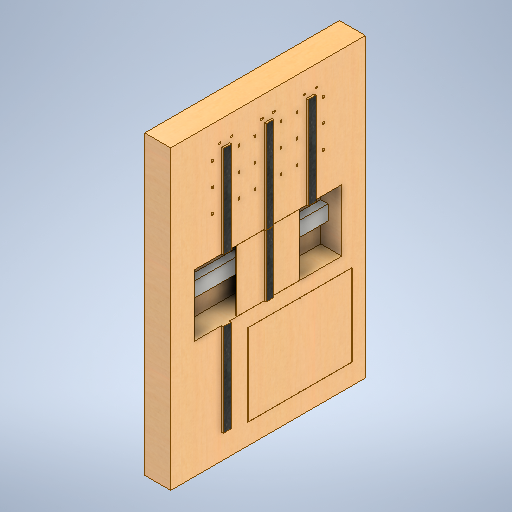
# Autodesk Inventor part: 3D cely
Saved by Autodesk Inventor 2025.1 (Build 291241000, 241)
## iProperties
Created: 2024-11-03
Part Number: 3D cely
Material: ABS plast
Document SubType Name: Sheet Metal
Designer: nelan
Density: 1.06 g/cm^3
Appearance: Borovice těžká – masiv světle obarvený – nízký lesk
Sheet Metal Rule: Výchozí
Author: nelan
Autodesk Inventor part; units mm, degrees
ref_plane "YZ Plane" through (0, 0, 0) normal (1, 0, 0) x (0, 1, 0)
ref_plane "XZ Plane" through (0, 0, 0) normal (0, 1, 0) x (-1, 0, 0)
ref_plane "XY Plane" through (0, 0, 0) normal (0, 0, 1) x (1, 0, 0)
sketch "Náčrt1" plane through (0, 0, 0) normal (1, 0, 0) x (0, 1, 0)
  line L0 (-400, -262.5) -> (400, -262.5)
  line L1 (400, -262.5) -> (400, 262.5)
  line L2 (-400, 262.5) -> (-400, -262.5)
  line L3 (-400, -262.5) -> (400, 262.5) construction
  line L4 (400, -262.5) -> (-400, 262.5) construction
  line L5 (-400, -262.5) -> (-320, -262.5)
  line L6 (-320, -262.5) -> (-320, -258.5)
  line L7 (-320, -258.5) -> (-400, -258.5)
  line L8 (-400, -258.5) -> (-400, -262.5)
  line L9 (-240, -258.5) -> (-240, -262.5)
  line L10 (-240, -258.5) -> (-160, -258.5)
  line L11 (-160, -258.5) -> (-160, -262.5)
  line L12 (-80, -258.5) -> (0, -258.5)
  line L13 (0, -258.5) -> (0, -262.5)
  line L14 (-80, -258.5) -> (-80, -262.5)
  line L15 (80, -258.5) -> (80, -262.5)
  line L16 (80, -258.5) -> (160, -258.5)
  line L17 (160, -258.5) -> (160, -262.5)
  line L18 (240, -258.5) -> (240, -262.5)
  line L19 (240, -258.5) -> (320, -258.5)
  line L20 (320, -258.5) -> (320, -262.5)
  line L21 (-400, 262.5) -> (400, 262.5)
  line L22 (-396, -258.5) -> (-400, -258.5)
  line L23 (-396, -258.5) -> (-400, -258.5)
  line L24 (-320, 258.5) -> (-240, 258.5)
  line L25 (-160, 258.5) -> (-80, 258.5)
  line L26 (0, 258.5) -> (80, 258.5)
  line L27 (160, 258.5) -> (240, 258.5)
  line L28 (320, 258.5) -> (400, 258.5)
  line L29 (320, 258.5) -> (320, 262.5)
  line L30 (240, 258.5) -> (240, 262.5)
  line L31 (160, 258.5) -> (160, 262.5)
  line L32 (80, 258.5) -> (80, 262.5)
  line L33 (0, 258.5) -> (0, 262.5)
  line L34 (-80, 258.5) -> (-80, 262.5)
  line L35 (-160, 258.5) -> (-160, 262.5)
  line L36 (-240, 258.5) -> (-240, 262.5)
  line L37 (-320, 258.5) -> (-320, 262.5)
  line L38 (400, 258.5) -> (396, 258.5)
  line L39 (396, 206.4) -> (396, 154.3)
  line L40 (396, 102.2) -> (396, 50.1)
  line L41 (396, -2) -> (396, -54.1)
  line L42 (396, -106.2) -> (396, -158.3)
  line L43 (396, -210.4) -> (396, -262.5)
  line L44 (-396, 262.5) -> (-396, 210.4)
  line L45 (-396, 210.4) -> (-400, 210.4)
  line L46 (-396, 158.3) -> (-396, 106.2)
  line L47 (-396, 54.1) -> (-396, 2)
  line L48 (-396, -50.1) -> (-396, -102.2)
  line L49 (-396, -154.3) -> (-396, -206.4)
  line L50 (-396, 158.3) -> (-400, 158.3)
  line L51 (-396, 106.2) -> (-400, 106.2)
  line L52 (-396, 54.1) -> (-400, 54.1)
  line L53 (-396, 2) -> (-400, 2)
  line L54 (-396, -50.1) -> (-400, -50.1)
  line L55 (-396, -102.2) -> (-400, -102.2)
  line L56 (-396, -154.3) -> (-400, -154.3)
  line L57 (-396, -206.4) -> (-400, -206.4)
  line L58 (396, 206.4) -> (400, 206.4)
  line L59 (396, 154.3) -> (400, 154.3)
  line L60 (396, 102.2) -> (400, 102.2)
  line L61 (396, 50.1) -> (400, 50.1)
  line L62 (396, -2) -> (400, -2)
  line L63 (396, -54.1) -> (400, -54.1)
  line L64 (396, -106.2) -> (400, -106.2)
  line L65 (396, -158.3) -> (400, -158.3)
  line L66 (396, -210.4) -> (400, -210.4)
  line L67 (396, -262.5) -> (400, -262.5)
  point P0 (0, 0)
  dimension "d0" = 800
  dimension "d1" = 525
  dimension "d4" = 80
  dimension "d5" = 4
  dimension "d7" = 80
  dimension "d9" = 80
  dimension "d11" = 80
  dimension "d13" = 80
  dimension "d14" = 4
  dimension "d15" = 4
  dimension "d16" = 4
  dimension "d17" = 4
  dimension "d18" = 4
  dimension "d19" = 4
  dimension "d20" = 80
  dimension "d21" = 80
  dimension "d22" = 80
  dimension "d40" = 80
  dimension "d41" = 80
  dimension "d42" = 80
  dimension "d43" = 80
  dimension "d44" = 80
  dimension "d45" = 80
  dimension "d46" = 80
  dimension "d47" = 80
  dimension "d48" = 80
  dimension "d49" = 4
  dimension "d50" = 4
  dimension "d51" = 52.1
  dimension "d52" = 52.1
  dimension "d53" = 52.1
  dimension "d54" = 52.1
  dimension "d55" = 52.1
  dimension "d56" = 52.1
  dimension "d57" = 52.1
  dimension "d58" = 52.1
  dimension "d59" = 52.1
  dimension "d60" = 52.1
  dimension "d67" = 52.1
  dimension "d68" = 52.1
  dimension "d69" = 52.1
  dimension "d70" = 52.1
  dimension "d71" = 52.1
  dimension "d72" = 52.1
  dimension "d73" = 52.1
  dimension "d74" = 52.1
  dimension "d75" = 52.1
  dimension "d76" = 52.1
  dimension "d77" = 4
  dimension "d78" = 4
  dimension "d79" = 4
  dimension "d80" = 4
  dimension "d81" = 4
  dimension "d82" = 4
  dimension "d83" = 4
  dimension "d84" = 4
  dimension "d85" = 4
  constraints: 128 end point, 20 horizontal, 16 vertical, 12 point on line, 9 vertical alignment, 6 horizontal alignment, 4 parallel, 2 midpoint, 2 perpendicular, 1 coincident, 50 other
  measures "d0" distance of L4.end L3.end
  measures "d1" distance of L3.end L4.start
  measures "d4" distance of L7.end L6.end
  measures "d5" distance of L6.end L5.end
  measures "d7" distance of L9.start L10.end
  measures "d9" distance of L12.start L12.end
  measures "d11" distance of L15.start L16.end
  measures "d13" distance of L18.start L19.end
  measures "d14" distance of L9.end L9.start
  measures "d15" distance of L11.end L10.end
  measures "d16" distance of L13.end L12.end
  measures "d17" distance of L17.end L16.end
  measures "d18" distance of L18.end L18.start
  measures "d19" distance of L20.end L19.end
  measures "d20" distance of L4.start L20.end
  measures "d21" distance of L18.end L17.end
  measures "d22" distance of L11.end L14.end
  measures "d40" distance of L24.start L24.end
  measures "d41" distance of L24.end L25.start
  measures "d42" distance of L25.start L25.end
  measures "d43" distance of L25.end L26.start
  measures "d44" distance of L26.start L26.end
  measures "d45" distance of L26.end L27.start
  measures "d46" distance of L27.start L27.end
  measures "d47" distance of L27.end L28.start
  measures "d48" distance of L28.start L28.end
  measures "d49" distance of L24.start L37.end
  measures "d50" distance of L28.end L38.end
  measures "d51" distance of L38.end L39.start
  measures "d52" distance of L39.start L39.end
  measures "d53" distance of L39.end L40.start
  measures "d54" distance of L40.start L40.end
  measures "d55" distance of L40.end L41.start
  measures "d56" distance of L41.start L41.end
  measures "d57" distance of L41.end L42.start
  measures "d58" distance of L42.start L42.end
  measures "d59" distance of L42.end L43.start
  measures "d60" distance of L43.start L43.end
  measures "d67" distance of L44.start L44.end
  measures "d68" distance of L44.end L46.start
  measures "d69" distance of L46.start L46.end
  measures "d70" distance of L46.end L47.start
  measures "d71" distance of L47.start L47.end
  measures "d72" distance of L47.end L48.start
  measures "d73" distance of L48.start L48.end
  measures "d74" distance of L48.end L49.start
  measures "d75" distance of L49.start L49.end
  measures "d76" distance of L49.end L22.start
  measures "d81" distance of L43.start L66.end
  measures "d82" distance of L42.end L65.end
  measures "d83" distance of L41.end L63.end
  measures "d84" distance of L40.end L61.end
  measures "d85" distance of L39.end L59.end
extrude "Vysunutí2" add sketch "Náčrt1" against normal blind 4 contours L6 L7 L2 L57 L49 L56 L55 L48 L54 L53 L47 L52 L51 L46 L50 L45 L44 L21 L37 L24 L36 L35 L25 L34 L33 L26 L32 L31 L27 L30 L29 L28 L1 L58 L39 L59 L60 L40 L61 L62 L41 L63 L64 L42 L65 L66 L43 L0 L20 L19 L18 L17 L16 L15 L13 L12 L14 L11 L10 L9
sketch "Náčrt4" plane through (0, -240, -258.5) normal (0, 0, -1) x (-1, 0, 0)
  line L0 (0, -160) -> (4, -160) projected
  line L1 (0, -160) -> (70, -160)
  line L2 (70, -160) -> (70, 640)
  line L3 (70, 640) -> (0, 640)
  line L4 (0, 640) -> (0, -160)
  line L5 (57, -64) -> (65, -64)
  line L6 (65, -64) -> (65, 16)
  line L7 (65, 16) -> (57, 16)
  line L8 (57, 16) -> (57, -64)
  line L9 (65, 112) -> (57, 112)
  line L10 (57, 112) -> (57, 192)
  line L11 (57, 192) -> (65, 192)
  line L12 (65, 192) -> (65, 112)
  line L13 (57, 288) -> (65, 288)
  line L14 (65, 288) -> (65, 368)
  line L15 (65, 368) -> (57, 368)
  line L16 (57, 368) -> (57, 288)
  line L17 (65, 544) -> (57, 544)
  line L18 (57, 544) -> (57, 464)
  line L19 (57, 464) -> (65, 464)
  line L20 (65, 464) -> (65, 544)
  point P0 (0, 240)
  dimension "d88" = 70
  dimension "d89" = 800
  dimension "d90" = 8
  dimension "d91" = 80
  dimension "d92" = 8
  dimension "d93" = 80
  dimension "d94" = 8
  dimension "d95" = 80
  dimension "d96" = 8
  dimension "d97" = 80
  dimension "d98" = 96
  dimension "d99" = 96
  dimension "d100" = 96
  dimension "d101" = 96
  dimension "d102" = 5
  dimension "d103" = 5
  dimension "d104" = 5
  constraints: 40 end point, 10 parallel, 5 horizontal, 5 perpendicular, 1 point on line
  measures "d88" distance of L3.end L2.end
  measures "d89" distance of L2.end L1.end
  measures "d90" distance of L7.end L6.end
  measures "d91" distance of L6.end L5.end
  measures "d92" distance of L10.end L11.end
  measures "d93" distance of L9.end L10.end
  measures "d94" distance of L15.end L14.end
  measures "d95" distance of L14.end L13.end
  measures "d96" distance of L19.end L18.end
  measures "d97" distance of L18.end L17.end
  measures "d98" vertical distance of L5.end L1.end
  measures "d99" vertical distance of L2.end L17.end
  measures "d100" distance of L18.end L15.end
  measures "d101" distance of L13.start L10.end
  measures "d102" distance between parallel lines of L2 L6
  measures "d103" distance between parallel lines of L2 L12
  measures "d104" distance between parallel lines of L2 L20
extrude "Vysunutí3" add sketch "Náčrt4" along normal blind 4
sketch "Náčrt5" plane through (0, -396, 2) normal (0, -1, 0) x (1, 0, 0)
  line L0 (-70, -260.5) -> (-70, -264.5) projected
  line L1 (0, 260.5) -> (-70, 260.5)
  line L2 (-70, 260.5) -> (-70, -264.5)
  line L3 (-70, -264.5) -> (0, -264.5)
  line L4 (0, -264.5) -> (0, 260.5)
  line L5 (-57, 187.25) -> (-65, 187.25)
  line L6 (-65, 187.25) -> (-65, 107.25)
  line L7 (-65, 107.25) -> (-57, 107.25)
  line L8 (-57, 107.25) -> (-57, 187.25)
  line L9 (-57, 40) -> (-65, 40)
  line L10 (-65, 40) -> (-65, -40)
  line L11 (-65, -40) -> (-57, -40)
  line L12 (-57, -40) -> (-57, 40)
  line L13 (-57, -111.25) -> (-65, -111.25)
  line L14 (-65, -111.25) -> (-65, -191.25)
  line L15 (-65, -191.25) -> (-57, -191.25)
  line L16 (-57, -191.25) -> (-57, -111.25)
  line L17 (0, 0) -> (-4, 0) projected
  line L18 (-4, -260.5) -> (-70, -260.5) projected
  point P0 (0, -2)
  point P1 (-57, 0)
  point P2 (-2, 0)
  dimension "d107" = 70
  dimension "d108" = 525
  dimension "d109" = 8
  dimension "d110" = 80
  dimension "d111" = 8
  dimension "d112" = 80
  dimension "d113" = 8
  dimension "d114" = 80
  dimension "d115" = 5
  dimension "d116" = 5
  dimension "d117" = 73.25
  dimension "d118" = 69.25
  constraints: 32 end point, 8 parallel, 4 horizontal, 4 perpendicular, 2 midpoint, 1 horizontal alignment, 1 point on line
  measures "d107" distance of L0.end L3.end
  measures "d108" distance of L1.end L0.end
  measures "d109" distance of L7.end L6.end
  measures "d110" distance of L6.end L5.end
  measures "d111" distance of L11.end L10.end
  measures "d112" distance of L10.end L9.end
  measures "d113" distance of L15.end L14.end
  measures "d114" distance of L14.end L13.end
  measures "d115" distance between parallel lines of L2 L10
  measures "d116" distance between parallel lines of L2 L6
  measures "d117" vertical distance of L5.start L1.end
  measures "d118" distance from line of L18 L15.end
mirror "Zrcadlit1" about plane through (0, 0, 0) normal (0, 0, 1) of "Vysunutí3"
extrude "Vysunutí4" add sketch "Náčrt5" along normal blind 4
mirror "Zrcadlit2" about plane through (0, 0, 0) normal (0, 1, 0) of "Vysunutí4"
sketch "Náčrt6" plane through (0, 0, 0) normal (1, 0, 0) x (0, 0, -1)
  line L0 (-199, 83.5) -> (199, 83.5)
  line L1 (199, 83.5) -> (199, -83.5)
  line L2 (199, -83.5) -> (-199, -83.5)
  line L3 (-199, -83.5) -> (-199, 83.5)
  line L4 (-199, 83.5) -> (199, -83.5) construction
  line L5 (199, 83.5) -> (-199, -83.5) construction
  point P0 (0, 0)
  dimension "d121" = 398
  dimension "d122" = 167
  constraints: 12 end point, 2 midpoint, 2 parallel, 1 horizontal, 1 perpendicular
  measures "d121" distance of L1.end L2.end
  measures "d122" distance of L0.end L1.end
extrude "Vysunutí5" cut sketch "Náčrt6" against normal blind 4
sketch "Náčrt7" plane through (0, 83.5, -199) normal (0, -1, 0) x (1, 0, 0)
  line L0 (-57, 0) -> (-4, 0)
  line L1 (-4, 398) -> (-57, 398)
  line L2 (-57, 398) -> (-57, 0)
  line L3 (-4, 398) -> (-4, 0)
  line L4 (-4, 457.5) -> (-4, -59.5) projected
  point P0 (0, 199)
  point P1 (-4, 199)
  point P2 (-4, 199)
  dimension "d128" = 398
  dimension "d129" = 53
  constraints: 8 end point, 2 midpoint, 1 horizontal, 1 horizontal alignment, 1 parallel, 1 perpendicular, 1 vertical, 1 vertical alignment
  measures "d128" distance of L1.start L0.end
  measures "d129" distance of L1.start L1.end
extrude "Vysunutí6" add sketch "Náčrt7" against normal blind 4
mirror "Zrcadlit3" about plane through (0, 0, 0) normal (0, 1, 0) of "Vysunutí6"
sketch "Náčrt8" plane through (0, -83.5, -199) normal (0, 0, 1) x (1, 0, 0)
  line L0 (0, -316.5) -> (0, 483.5) projected
  line L1 (0, 167) -> (-57, 167)
  line L2 (-57, 167) -> (-57, 0)
  line L3 (-57, 0) -> (0, 0)
  line L4 (0, 83.5) -> (0, 0)
  line L5 (0, 83.5) -> (0, 0)
  line L6 (0, 167) -> (0, 0)
  point P0 (0, 83.5)
  dimension "d133" = 167
  dimension "d134" = 57
  constraints: 12 end point, 3 collinear, 2 horizontal alignment, 2 midpoint, 2 perpendicular, 2 point on line, 1 coincident, 1 vertical alignment
  measures "d133" distance of L3.end L1.start
  measures "d134" distance of L1.start L1.end
extrude "Vysunutí7" add sketch "Náčrt8" against normal blind 4
mirror "Zrcadlit4" about plane through (0, 0, 0) normal (0, 0, 1) of "Vysunutí7"
sketch "Náčrt10" plane through (-57, -87.5, -199) normal (-1, 0, 0) x (0, 0, 1)
  line L0 (-63.5, -312.5) -> (-63.5, 487.5) projected
  line L1 (461.5, -312.5) -> (-63.5, -312.5)
  line L2 (-63.5, -312.5) -> (-63.5, 487.5)
  line L3 (-63.5, 487.5) -> (461.5, 487.5)
  line L4 (461.5, 487.5) -> (461.5, -312.5)
  line L5 (461.5, -312.5) -> (-63.5, 487.5) construction
  line L6 (-63.5, -312.5) -> (461.5, 487.5) construction
  point P0 (199, 87.5)
  constraints: 12 end point, 2 midpoint, 2 parallel, 1 horizontal, 1 perpendicular
extrude "Vysunutí8" add sketch "Náčrt10" along normal blind 8
sketch "Náčrt11" plane through (-57, -87.5, -199) normal (1, 0, 0) x (0, 0, -1)
  line L0 (-398, 107.5) -> (0, 107.5)
  line L1 (0, 107.5) -> (0, 67.5)
  line L2 (0, 67.5) -> (-398, 67.5)
  line L3 (-398, 67.5) -> (-398, 107.5)
  line L4 (-398, 107.5) -> (0, 67.5) construction
  line L5 (0, 107.5) -> (-398, 67.5) construction
  point P0 (-199, 87.5)
  dimension "d139" = 398
  dimension "d140" = 40
  constraints: 12 end point, 2 midpoint, 2 parallel, 1 horizontal, 1 perpendicular
  measures "d139" distance of L1.end L2.end
  measures "d140" distance of L0.end L1.end
extrude "Vysunutí9" add sketch "Náčrt11" along normal blind 20
sketch "Náčrt12" plane through (-37, -87.5, -199) normal (1, 0, 0) x (0, 0, -1)
  line L0 (-234, 132.5) -> (-164, 132.5)
  line L1 (-164, 132.5) -> (-164, 42.5)
  line L2 (-164, 42.5) -> (-234, 42.5)
  line L3 (-234, 42.5) -> (-234, 132.5)
  line L4 (-234, 132.5) -> (-164, 42.5) construction
  line L5 (-164, 132.5) -> (-234, 42.5) construction
  point P0 (-199, 87.5)
  dimension "d143" = 70
  dimension "d144" = 90
  constraints: 12 end point, 2 midpoint, 2 parallel, 1 horizontal, 1 perpendicular
  measures "d143" distance of L1.end L2.end
  measures "d144" distance of L0.end L1.end
extrude "Vysunutí10" add sketch "Náčrt12" along normal blind 33
sketch "Náčrt13" plane through (-4, -87.5, -199) normal (1, 0, 0) x (0, 0, -1)
  line L0 (-282.75, 170.5) -> (-115.25, 170.5)
  line L1 (-115.25, 170.5) -> (-115.25, 4.5)
  line L2 (-115.25, 4.5) -> (-282.75, 4.5)
  line L3 (-282.75, 4.5) -> (-282.75, 170.5)
  line L4 (-282.75, 170.5) -> (-115.25, 4.5) construction
  line L5 (-115.25, 170.5) -> (-282.75, 4.5) construction
  point P0 (-199, 87.5)
  dimension "d147" = 167.5
  dimension "d148" = 166
  constraints: 12 end point, 2 midpoint, 2 parallel, 1 horizontal, 1 perpendicular
  measures "d147" distance of L1.end L2.end
  measures "d148" distance of L0.end L1.end
extrude "Vysunutí11" add sketch "Náčrt13" along normal blind 4
sketch "Náčrt14" plane through (0, 0, 0) normal (1, 0, 0) x (0, 0, -1)
  line L0 (-199, -83.5) -> (199, -83.5) projected
  line L1 (-104.75, -83.5) -> (-104.75, -249.5)
  line L2 (-104.75, -249.5) -> (-125.75, -249.5)
  line L3 (-125.75, -249.5) -> (-125.75, -83.5)
  line L4 (-104.75, -249.5) -> (-104.75, -332.5)
  line L5 (-104.75, -332.5) -> (-125.75, -332.5)
  line L6 (-125.75, -332.5) -> (-125.75, -249.5)
  line L7 (83.75, 83) -> (-83.75, 83) projected
  line L8 (-10.5, 83) -> (-10.5, -83.5)
  line L9 (10.5, -83.5) -> (10.5, 83)
  line L10 (-10.5, -0.25) -> (10.5, -0.25)
  line L11 (-103.5, 332.5) -> (-103.5, 166.5)
  line L12 (-103.5, 166.5) -> (-124.5, 166.5)
  line L13 (-124.5, 166.5) -> (-124.5, 332.5)
  line L14 (-103.5, 166.5) -> (-103.5, 83.5)
  line L15 (-103.5, 83.5) -> (-124.5, 83.5)
  line L16 (-124.5, 83.5) -> (-124.5, 166.5)
  line L17 (-199, 83.5) -> (199, 83.5) projected
  line L18 (-124.5, 332.5) -> (-103.5, 332.5)
  line L19 (-10.5, 83.5) -> (10.5, 83.5)
  line L20 (10.5, 83.5) -> (10.5, 166.5)
  line L21 (10.5, 166.5) -> (-10.5, 166.5)
  line L22 (-10.5, 166.5) -> (-10.5, 83.5)
  line L23 (-10.5, 166.5) -> (-10.5, 332.5)
  line L24 (-10.5, 332.5) -> (10.5, 332.5)
  line L25 (10.5, 332.5) -> (10.5, 166.5)
  line L26 (103.5, 83.5) -> (103.5, 166.5)
  line L27 (103.5, 166.5) -> (124.5, 166.5)
  line L28 (124.5, 166.5) -> (124.5, 83.5)
  line L29 (103.5, 83.5) -> (124.5, 83.5)
  line L30 (103.5, 166.5) -> (103.5, 332.5)
  line L31 (103.5, 332.5) -> (124.5, 332.5)
  line L32 (124.5, 332.5) -> (124.5, 166.5)
  point P0 (0, 0)
  point P1 (0, -0.25)
  point P2 (-114, 83.5)
  point P3 (0, 83.5)
  point P4 (0, 83.5)
  point P5 (0, 166.5)
  point P6 (114, 83.5)
  point P7 (0, 83.5)
  point P8 (114, 166.5)
  dimension "d151" = 166
  dimension "d153" = 21
  dimension "d154" = 73.25
  dimension "d155" = 83
  dimension "d156" = 21
  dimension "d157" = 166
  dimension "d158" = 21
  dimension "d159" = 83
  dimension "d160" = 74.5
  dimension "d161" = 166
  dimension "d162" = 21
  dimension "d163" = 83
  dimension "d164" = 166
  dimension "d165" = 83
  dimension "d166" = 21
  dimension "d167" = 74.5
  constraints: 60 end point, 17 point on line, 16 perpendicular, 10 midpoint, 5 vertical, 3 collinear, 3 vertical alignment, 2 horizontal alignment, 1 parallel
  measures "d151" distance of L2.end L3.end
  measures "d153" distance between parallel lines of L1 L3
  measures "d154" distance from line of L0.start L3
  measures "d155" distance of L1.end L4.end
  measures "d156" distance between parallel lines of L9 L8
  measures "d157" distance of L12.end L13.end
  measures "d158" distance between parallel lines of L11 L13
  measures "d159" distance of L11.end L14.end
  measures "d160" distance of L15.end L17.start
  measures "d161" distance of L24.end L20.end
  measures "d162" distance of L23.end L24.end
  measures "d163" distance of L19.end L20.end
  measures "d164" distance of L31.end L27.end
  measures "d165" distance of L27.end L28.end
  measures "d166" distance of L30.end L31.end
  measures "d167" distance from line of L17.end L28
extrude "Vysunutí12" add sketch "Náčrt14" along normal blind 5
sketch "Náčrt16" plane through (0, 0, 0) normal (1, 0, 0) x (0, 0, -1)
  line L0 (-151.5, 316.5) -> (-151.5, 310.5)
  line L1 (-151.5, 310.5) -> (-147.5, 310.5)
  line L2 (-147.5, 310.5) -> (-147.5, 316.5)
  line L3 (-147.5, 316.5) -> (-151.5, 316.5)
  line L4 (-151.5, 254.5) -> (-151.5, 248.5)
  line L5 (-151.5, 248.5) -> (-147.5, 248.5)
  line L6 (-147.5, 248.5) -> (-147.5, 254.5)
  line L7 (-147.5, 254.5) -> (-151.5, 254.5)
  line L8 (-151.5, 192.5) -> (-151.5, 186.5)
  line L9 (-151.5, 186.5) -> (-147.5, 186.5)
  line L10 (-147.5, 186.5) -> (-147.5, 192.5)
  line L11 (-147.5, 192.5) -> (-151.5, 192.5)
  line L12 (-80.5, 316.5) -> (-80.5, 310.5)
  line L13 (-80.5, 310.5) -> (-76.5, 310.5)
  line L14 (-76.5, 310.5) -> (-76.5, 316.5)
  line L15 (-76.5, 316.5) -> (-80.5, 316.5)
  line L16 (-80.5, 254.5) -> (-80.5, 248.5)
  line L17 (-80.5, 248.5) -> (-76.5, 248.5)
  line L18 (-76.5, 248.5) -> (-76.5, 254.5)
  line L19 (-76.5, 254.5) -> (-80.5, 254.5)
  line L20 (-80.5, 192.5) -> (-80.5, 186.5)
  line L21 (-80.5, 186.5) -> (-76.5, 186.5)
  line L22 (-76.5, 186.5) -> (-76.5, 192.5)
  line L23 (-76.5, 192.5) -> (-80.5, 192.5)
  line L24 (-37.5, 316.5) -> (-37.5, 310.5)
  line L25 (-37.5, 310.5) -> (-33.5, 310.5)
  line L26 (-33.5, 310.5) -> (-33.5, 316.5)
  line L27 (-33.5, 316.5) -> (-37.5, 316.5)
  line L28 (-37.5, 254.5) -> (-37.5, 248.5)
  line L29 (-37.5, 248.5) -> (-33.5, 248.5)
  line L30 (-33.5, 248.5) -> (-33.5, 254.5)
  line L31 (-33.5, 254.5) -> (-37.5, 254.5)
  line L32 (-37.5, 192.5) -> (-37.5, 186.5)
  line L33 (-37.5, 186.5) -> (-33.5, 186.5)
  line L34 (-33.5, 186.5) -> (-33.5, 192.5)
  line L35 (-33.5, 192.5) -> (-37.5, 192.5)
  line L36 (33.5, 316.5) -> (33.5, 310.5)
  line L37 (33.5, 310.5) -> (37.5, 310.5)
  line L38 (37.5, 310.5) -> (37.5, 316.5)
  line L39 (37.5, 316.5) -> (33.5, 316.5)
  line L40 (33.5, 254.5) -> (33.5, 248.5)
  line L41 (33.5, 248.5) -> (37.5, 248.5)
  line L42 (37.5, 248.5) -> (37.5, 254.5)
  line L43 (37.5, 254.5) -> (33.5, 254.5)
  line L44 (33.5, 192.5) -> (33.5, 186.5)
  line L45 (33.5, 186.5) -> (37.5, 186.5)
  line L46 (37.5, 186.5) -> (37.5, 192.5)
  line L47 (37.5, 192.5) -> (33.5, 192.5)
  line L48 (76.5, 316.5) -> (76.5, 310.5)
  line L49 (76.5, 310.5) -> (80.5, 310.5)
  line L50 (80.5, 310.5) -> (80.5, 316.5)
  line L51 (80.5, 316.5) -> (76.5, 316.5)
  line L52 (76.5, 254.5) -> (76.5, 248.5)
  line L53 (76.5, 248.5) -> (80.5, 248.5)
  line L54 (80.5, 248.5) -> (80.5, 254.5)
  line L55 (80.5, 254.5) -> (76.5, 254.5)
  line L56 (76.5, 192.5) -> (76.5, 186.5)
  line L57 (76.5, 186.5) -> (80.5, 186.5)
  line L58 (80.5, 186.5) -> (80.5, 192.5)
  line L59 (80.5, 192.5) -> (76.5, 192.5)
  line L60 (147.5, 316.5) -> (147.5, 310.5)
  line L61 (147.5, 310.5) -> (151.5, 310.5)
  line L62 (151.5, 310.5) -> (151.5, 316.5)
  line L63 (151.5, 316.5) -> (147.5, 316.5)
  line L64 (147.5, 254.5) -> (147.5, 248.5)
  line L65 (147.5, 248.5) -> (151.5, 248.5)
  line L66 (151.5, 248.5) -> (151.5, 254.5)
  line L67 (151.5, 254.5) -> (147.5, 254.5)
  line L68 (147.5, 192.5) -> (147.5, 186.5)
  line L69 (147.5, 186.5) -> (151.5, 186.5)
  line L70 (151.5, 186.5) -> (151.5, 192.5)
  line L71 (151.5, 192.5) -> (147.5, 192.5)
  line L72 (-103.5, 83.5) -> (-103.5, 332.5) projected
  line L73 (-10.5, 83.5) -> (-10.5, 332.5) projected
  line L74 (10.5, 83.5) -> (10.5, 332.5) projected
  line L75 (103.5, 83.5) -> (103.5, 332.5) projected
  line L76 (124.5, 83.5) -> (124.5, 332.5) projected
  line L77 (-124.5, 332.5) -> (-124.5, 83.5) projected
  line L78 (-133.17, 346.5) -> (-133.17, 342.5)
  line L79 (-133.17, 342.5) -> (-127.17, 342.5)
  line L80 (-127.17, 342.5) -> (-127.17, 346.5)
  line L81 (-127.17, 346.5) -> (-133.17, 346.5)
  line L82 (-100.83, 346.5) -> (-100.83, 342.5)
  line L83 (-100.83, 342.5) -> (-94.83, 342.5)
  line L84 (-94.83, 342.5) -> (-94.83, 346.5)
  line L85 (-94.83, 346.5) -> (-100.83, 346.5)
  line L86 (-19.17, 346.5) -> (-19.17, 342.5)
  line L87 (-19.17, 342.5) -> (-13.17, 342.5)
  line L88 (-13.17, 342.5) -> (-13.17, 346.5)
  line L89 (-13.17, 346.5) -> (-19.17, 346.5)
  line L90 (13.17, 346.5) -> (13.17, 342.5)
  line L91 (13.17, 342.5) -> (19.17, 342.5)
  line L92 (19.17, 342.5) -> (19.17, 346.5)
  line L93 (19.17, 346.5) -> (13.17, 346.5)
  line L94 (94.83, 346.5) -> (94.83, 342.5)
  line L95 (94.83, 342.5) -> (100.83, 342.5)
  line L96 (100.83, 342.5) -> (100.83, 346.5)
  line L97 (100.83, 346.5) -> (94.83, 346.5)
  line L98 (127.17, 346.5) -> (127.17, 342.5)
  line L99 (127.17, 342.5) -> (133.17, 342.5)
  line L100 (133.17, 342.5) -> (133.17, 346.5)
  line L101 (133.17, 346.5) -> (127.17, 346.5)
  point P0 (0, 0)
  point P1 (-37.5, 313.5)
  point P2 (37.5, 313.5)
  dimension "d171" = 4
  dimension "d172" = 16
  dimension "d173" = 6
  dimension "d175" = 56
  dimension "d176" = 6
  dimension "d177" = 4
  dimension "d178" = 6
  dimension "d179" = 4
  dimension "d180" = 56
  dimension "d181" = 4
  dimension "d182" = 6
  dimension "d183" = 56
  dimension "d184" = 6
  dimension "d185" = 4
  dimension "d186" = 6
  dimension "d187" = 4
  dimension "d188" = 56
  dimension "d189" = 4
  dimension "d190" = 6
  dimension "d191" = 56
  dimension "d192" = 6
  dimension "d193" = 4
  dimension "d194" = 6
  dimension "d195" = 4
  dimension "d196" = 56
  dimension "d197" = 4
  dimension "d198" = 6
  dimension "d199" = 56
  dimension "d200" = 6
  dimension "d201" = 4
  dimension "d202" = 6
  dimension "d203" = 4
  dimension "d204" = 56
  dimension "d205" = 4
  dimension "d206" = 6
  dimension "d207" = 56
  dimension "d208" = 6
  dimension "d209" = 4
  dimension "d210" = 6
  dimension "d211" = 4
  dimension "d212" = 56
  dimension "d213" = 4
  dimension "d214" = 6
  dimension "d215" = 56
  dimension "d216" = 6
  dimension "d217" = 4
  dimension "d218" = 6
  dimension "d219" = 4
  dimension "d220" = 56
  dimension "d228" = 27
  dimension "d229" = 27
  dimension "d230" = 27
  dimension "d231" = 27
  dimension "d232" = 27
  dimension "d233" = 27
  dimension "d246" = 4
  dimension "d247" = 6
  dimension "d248" = 4
  dimension "d249" = 6
  dimension "d254" = 18.33
  dimension "d255" = 18.33
  dimension "d256" = 26
  dimension "d259" = 4
  dimension "d260" = 6
  constraints: 192 end point, 63 perpendicular, 21 vertical, 12 point on line, 12 vertical alignment, 6 parallel, 5 horizontal alignment, 2 midpoint
  measures "d171" distance of L2.end L0.start
  measures "d172" vertical distance of L77.start L2.end
  measures "d173" distance of L1.end L2.end
  measures "d175" distance of L1.end L6.end
  measures "d176" distance of L5.end L6.end
  measures "d177" distance of L6.end L4.start
  measures "d178" distance of L9.end L10.end
  measures "d179" distance of L10.end L8.start
  measures "d180" distance of L10.end L5.end
  measures "d181" distance of L15.start L15.end
  measures "d182" distance of L13.end L15.start
  measures "d183" distance of L13.end L19.start
  measures "d184" distance of L17.end L19.start
  measures "d185" distance of L19.start L19.end
  measures "d186" distance of L21.end L23.start
  measures "d187" distance of L23.start L23.end
  measures "d188" distance of L23.start L17.end
  measures "d189" distance of L27.start L27.end
  measures "d190" distance of L25.end L27.start
  measures "d191" distance of L25.end L31.start
  measures "d192" distance of L29.end L31.start
  measures "d193" distance of L31.start L31.end
  measures "d194" distance of L33.end L35.start
  measures "d195" distance of L35.start L35.end
  measures "d196" distance of L35.start L29.end
  measures "d197" distance of L39.start L39.end
  measures "d198" distance of L37.end L39.start
  measures "d199" distance of L37.end L43.start
  measures "d200" distance of L41.end L43.start
  measures "d201" distance of L43.start L43.end
  measures "d202" distance of L45.end L47.start
  measures "d203" distance of L47.start L47.end
  measures "d204" distance of L47.start L41.end
  measures "d205" distance of L51.start L51.end
  measures "d206" distance of L49.end L51.start
  measures "d207" distance of L49.end L55.start
  measures "d208" distance of L53.end L55.start
  measures "d209" distance of L55.start L55.end
  measures "d210" distance of L57.end L59.start
  measures "d211" distance of L59.start L59.end
  measures "d212" distance of L59.start L53.end
  measures "d213" distance of L63.start L63.end
  measures "d214" distance of L61.end L63.start
  measures "d215" distance of L61.end L67.start
  measures "d216" distance of L65.end L67.start
  measures "d217" distance of L67.start L67.end
  measures "d218" distance of L69.end L71.start
  measures "d219" distance of L71.start L71.end
  measures "d220" distance of L71.start L65.end
  measures "d228" distance from line of L77 L0.end
  measures "d229" distance from line of L72 L13.end
  measures "d230" distance from line of L73 L24.end
  measures "d231" distance from line of L74 L37.end
  measures "d232" distance from line of L75 L48.end
  measures "d233" distance from line of L61.end L76
  measures "d246" distance of L78.start L78.end
  measures "d247" distance of L78.end L79.end
  measures "d248" distance of L82.start L82.end
  measures "d249" distance of L82.end L83.end
  measures "d254" horizontal distance of L78.start L0.start
  measures "d255" horizontal distance of L15.start L84.end
  measures "d256" distance from line of L79 L2.end
  measures "d259" distance of L89.end L87.start
  measures "d260" distance of L87.start L87.end
extrude "Vysunutí13" cut sketch "Náčrt16" against normal blind 4 contours L3 L2 L1 L0 | L7 L6 L5 L4 | L11 L10 L9 L8 | L15 L14 L13 L12 | L19 L18 L17 L16 | L23 L22 L21 L20 | L27 L26 L25 L24 | L31 L30 L29 L28 | L35 L34 L33 L32 | L39 L38 L37 L36 | L43 L42 L41 L40 | L47 L46 L45 L44 | L51 L50 L49 L48 | L55 L54 L53 L52 | L59 L58 L57 L56 | L63 L62 L61 L60 | L67 L66 L65 L64 | L71 L70 L69 L68
sketch "Náčrt17" plane through (0, 0, 0) normal (1, 0, 0) x (0, 0, -1)
  line L0 (-54, -124.5) -> (226, -124.5)
  line L1 (226, -124.5) -> (226, -344.5)
  line L2 (226, -344.5) -> (-54, -344.5)
  line L3 (-54, -344.5) -> (-54, -124.5)
  line L4 (-54, -124.5) -> (226, -344.5) construction
  line L5 (226, -124.5) -> (-54, -344.5) construction
  line L6 (-54.5, -124) -> (226.5, -124)
  line L7 (226.5, -124) -> (226.5, -345)
  line L8 (226.5, -345) -> (-54.5, -345)
  line L9 (-54.5, -345) -> (-54.5, -124)
  line L10 (-54.5, -124) -> (226.5, -345) construction
  line L11 (226.5, -124) -> (-54.5, -345) construction
  arc A0 (83.4703, -124.5) -> (88.5297, -124.5) centre (86, -123.4174) ccw
  line L12 (262.5, -400) -> (262.5, 400) projected
  line L13 (262.5, -400) -> (-262.5, -400) projected
  arc A1 (88.6895, -344.5) -> (83.3105, -344.5) centre (86, -345.0833) ccw
  point P0 (0, 0)
  point P1 (86, -234.5)
  point P2 (86, -124.5)
  point P3 (86, -126.169)
  point P4 (86, -124)
  point P5 (86, -344.5)
  point P6 (86, -342.3313)
  dimension "d234" = 280
  dimension "d235" = 220
  dimension "d236" = 281
  dimension "d237" = 221
  dimension "d238" = 36
  dimension "d239" = 55
  dimension "d240" = 2.7516
  dimension "d241" = 2.169
  dimension "d242" = 2.752
  dimension "d243" = 2.1687
  constraints: 24 end point, 7 midpoint, 6 point on circle, 4 parallel, 4 point on line, 2 centre point, 2 horizontal, 2 perpendicular, 2 vertical alignment, 1 horizontal alignment
  measures "d234" distance of L1.end L2.end
  measures "d235" distance of L0.end L1.end
  measures "d236" distance of L7.end L8.end
  measures "d237" distance of L6.end L7.end
  measures "d238" distance between parallel lines of L12 L7
  measures "d239" distance between parallel lines of L13 L8
  measures "d240" radius of A0
  measures "d241" distance of point (86, -126.169) point (86, -124)
  measures "d242" radius of A1
  measures "d243" distance of point (86, -344.5) point (86, -342.331)
extrude "Vysunutí14" cut sketch "Náčrt17" against normal blind 4 contours L0 A0 | A1 L2 | L6 L7 L8 L9
extrude "Vysunutí15" cut sketch "Náčrt16" against normal blind 4 contours L81 L80 L79 L78 | L85 L84 L83 L82 | L89 L88 L87 L86 | L93 L92 L91 L90 | L97 L96 L95 L94 | L101 L100 L99 L98
